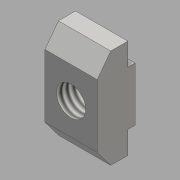
# Autodesk Inventor part: RHOMBUS NUT 4
Saved by Autodesk Inventor 2016 (Build 200138000, 138)
## iProperties
Created: 2023-12-25
Part Number: RHOMBUS NUT 4
Material: Generic
Document SubType Name: Modeling
Designer: Riskinova Oktavia
Density: 1 g/cm^3
Appearance: Default
Author: Riskinova Oktavia
Autodesk Inventor part; units mm, degrees
ref_plane "YZ Plane" through (0, 0, 0) normal (1, 0, 0) x (0, 1, 0)
ref_plane "XZ Plane" through (0, 0, 0) normal (0, 1, 0) x (-1, 0, 0)
ref_plane "XY Plane" through (0, 0, 0) normal (0, 0, 1) x (1, 0, 0)
sketch "Sketch1" plane through (0, 0, 0) normal (0, 1, 0) x (-1, 0, 0)
  line L0 (-2.9, 5.5) -> (2.9, 5.5)
  line L1 (2.9, 5.5) -> (2.9, -5.5)
  line L2 (2.9, -5.5) -> (-2.9, -5.5)
  line L3 (-2.9, -5.5) -> (-2.9, 5.5)
  line L4 (-2.9, 5.5) -> (2.9, -5.5) construction
  line L5 (2.9, 5.5) -> (-2.9, -5.5) construction
  point P0 (0, 0)
  dimension "d0" = 11
  dimension "d1" = 5.8
  constraints: 12 end point, 2 midpoint, 2 parallel, 1 horizontal, 1 perpendicular
  measures "d0" distance of L0.end L1.end
  measures "d1" distance of L1.end L2.end
extrude "Extrusion1" add sketch "Sketch1" along normal mid plane 4.2
sketch "Sketch2" plane through (2.9, -2.1, -5.5) normal (1, 0, 0) x (0, 0, -1)
  line L0 (0, 4.2) -> (0, 0) projected
  line L1 (-11, 4.2) -> (0, 4.2) projected
  line L2 (-11, 0) -> (-11, 4.2) projected
  line L3 (0, 0) -> (-11, 0) projected
  line L4 (-11, 0) -> (-11, 4.2) projected
  line L5 (-11, 1.5) -> (-9, 0)
  line L6 (0, 0) -> (-11, 0) projected
  line L7 (-2, 0) -> (0, 1.5)
  line L8 (-11, 4.2) -> (-8.5, 4.2)
  line L9 (-8.5, 4.2) -> (-8.5, 3.4)
  line L10 (-8.5, 3.4) -> (-11, 3.4)
  line L11 (-11, 3.4) -> (-11, 4.2)
  line L12 (0, 4.2) -> (-2.5, 4.2)
  line L13 (-2.5, 4.2) -> (-2.5, 3.4)
  line L14 (-2.5, 3.4) -> (0, 3.4)
  line L15 (0, 3.4) -> (0, 4.2)
  point P0 (-5.5, 2.1)
  dimension "d4" = 6
  dimension "d5" = 3
  dimension "d6" = 7
  dimension "d7" = 3.5
  dimension "d8" = 1.5
  dimension "d9" = 3.4
  constraints: 20 end point, 5 point on line, 4 collinear, 4 parallel, 2 horizontal, 2 perpendicular, 1 horizontal alignment
  measures "d4" distance between parallel lines of L13 L9
  measures "d5" distance from line of point (-5.5, 2.1) L9
  measures "d6" distance of L7.start L5.end
  measures "d7" horizontal distance of point (-5.5, 2.1) L5.end
  measures "d8" distance from line of L5.start L3
  measures "d9" distance between parallel lines of L3 L14
extrude "Extrusion2" cut sketch "Sketch2" against normal through all contours L0 L14 L13 L1 | L0 L3 L7 | L9 L10 L2 L1 | L3 L2 L5
sketch "Sketch3" plane through (0, 2.1, 0) normal (0, 1, 0) x (1, 0, 0)
  point P0 (0, 0)
  point P1 (0, 0)
  constraints: 1 coincident
hole "Hole1" at (0, 2.1, 0) direction (0, -1, 0) diameter 3.242 end through all thread size "M4x0.7" class "6H" standard "ISO Metric profile"
equation "\"d5\" = 0.5 * d4"
equation "\"d7\" = 0.5 * d6"
body "Solid1"
